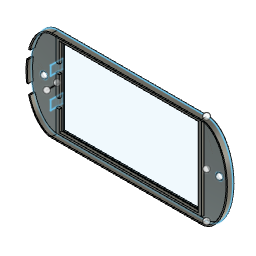
SolarPanelFront_v1 (Autodesk Fusion 360 design; units mm, degrees)
Autodesk Fusion 360 part; units mm, degrees
sketch "Sketch1" plane through (0, 0, 0) normal (0, 1, 0) x (1, 0, 0)
  line L0 (0, 0) -> (115, 0)
  line L1 (115, -70) -> (0, -70)
  ellipse E0 centre (0, -35) end of major axis (0, -70) minor radius 20 (0, 0) -> (0, -70) ccw
  ellipse E1 centre (115, -35) end of major axis (115, -70) minor radius 20 (115, -70) -> (115, 0) ccw
  circle A0 centre (-10, -35) radius 2.5
  circle A1 centre (125, -35) radius 2.5
  dimension "d1" = 20
  dimension "d2" = 5
  dimension "d3" = 10
  constraint horizontal L0
  constraint horizontal L1
  measures "d2" diameter of A0
  measures "d3" distance of E0.centre A0.centre
extrude "Extrude1" add sketch "Sketch1" along normal blind 1
sketch "Sketch3" plane through (0, 0, 0) normal (0, -1, 0) x (1, 0, 0)
  circle A0 centre (-10, 35) radius 2.5
  circle A1 centre (125, 35) radius 2.5
  ellipse E0 centre (0, 35) end of major axis (0, 70) minor radius 20 (0, 70) -> (0, 0) ccw
  line L0 (0, 0) -> (115, 0)
  ellipse E1 centre (115, 35) end of major axis (115, 70) minor radius 20 (115, 0) -> (115, 70) ccw
  line L1 (115, 70) -> (0, 70)
  line L2 (0, 1) -> (115, 1)
  spline S0 degree 3 poles (115, 1) (118.1745, 1) (121.3862, 2.4713) (124.2603, 5.3633) (127.2867, 8.4088) (129.8847, 13.0253) (131.6024, 18.5351) (133.5298, 24.7176) (134.3377, 31.9986) (133.8651, 39.0248) (133.4191, 45.6553) (131.8372, 52.0318) (129.4075, 57.0895) (127.2109, 61.662) (124.3332, 65.1363) (121.2436, 67.0835) (119.2133, 68.3631) (117.1029, 69) (115, 69) knots 3.141593 3.141593 3.141593 3.141593 3.663435 3.663435 3.663435 4.212955 4.212955 4.212955 4.82957 4.82957 4.82957 5.411454 5.411454 5.411454 5.937501 5.937501 5.937501 6.283185 6.283185 6.283185 6.283185
  line L3 (115, 69) -> (0, 69)
  spline S1 degree 3 poles (0, 69) (-3.1745, 69) (-6.3862, 67.5287) (-9.2603, 64.6367) (-12.2867, 61.5912) (-14.8847, 56.9747) (-16.6024, 51.4649) (-18.5298, 45.2824) (-19.3377, 38.0014) (-18.8651, 30.9752) (-18.4191, 24.3447) (-16.8372, 17.9682) (-14.4075, 12.9105) (-12.2109, 8.338) (-9.3332, 4.8637) (-6.2436, 2.9165) (-4.2133, 1.6369) (-2.1029, 1) (0, 1) knots 0 0 0 0 0.521842 0.521842 0.521842 1.071362 1.071362 1.071362 1.687978 1.687978 1.687978 2.269861 2.269861 2.269861 2.795908 2.795908 2.795908 3.141593 3.141593 3.141593 3.141593
  dimension "d6" = -1
extrude "Extrude2" add sketch "Sketch3" along normal blind 4 contours E0 L0 E1 L1
sketch "Sketch4" plane through (0, 0, 0) normal (0, 1, 0) x (1, 0, 0)
  line L0 (3.55, -65.5) -> (110.65, -65.5)
  line L1 (110.65, -65.5) -> (110.65, -4.5)
  line L2 (110.65, -4.5) -> (3.55, -4.5)
  line L3 (3.55, -4.5) -> (3.55, -65.5)
  line L4 (115, -1) -> (0, -1)
  line L5 (1, -67) -> (113, -67)
  line L6 (113, -67) -> (113, -3)
  line L7 (113, -3) -> (1, -3)
  line L8 (1, -3) -> (1, -67)
  point P0 (0, -35)
  dimension "d9" = 61
  dimension "d10" = 107.1
  dimension "d11" = 3.55
  dimension "d12" = 3.5
  constraint horizontal L0
  constraint vertical L1
  constraint horizontal L2
  constraint vertical L3
  constraint horizontal L5
  constraint vertical L6
  constraint horizontal L7
  constraint vertical L8
  measures "d9" distance of L0.start L2.end
  measures "d10" distance of L0.start L0.end
  measures "d11" distance of L3 P0
  measures "d12" distance of L2 L4
extrude "Extrude3" add sketch "Sketch4" against normal blind 2
sketch "Sketch5" plane through (0, 0, 0) normal (0, 1, 0) x (-1, 0, 0)
  line L0 (-4.5848, 64.4333) -> (-109.4505, 64.4333)
  line L1 (-109.4505, 64.4333) -> (-109.4505, 5.2457)
  line L2 (-109.4505, 5.2457) -> (-4.5848, 5.2457)
  line L3 (-4.5848, 5.2457) -> (-4.5848, 64.4333)
  constraint horizontal L0
  constraint vertical L1
  constraint horizontal L2
  constraint vertical L3
extrude "Extrude4" cut sketch "Sketch5" along normal blind 10
sketch "Sketch6" plane through (1, 0, 0) normal (-1, 0, 0) x (0, -1, 0)
  line L0 (0, 67) -> (0, 3)
  line L1 (0, 3) -> (2, 3)
  line L2 (2, 3) -> (2, 67)
  line L3 (2, 67) -> (0, 67)
  line L4 (-3, 27) -> (6, 27)
  line L5 (6, 27) -> (6, 20)
  line L6 (6, 20) -> (-3, 20)
  line L7 (-3, 20) -> (-3, 27)
  line L8 (0, 35) -> (9, 35)
  line L9 (-3, 43) -> (6, 43)
  line L10 (6, 43) -> (6, 50)
  line L11 (6, 50) -> (-3, 50)
  line L12 (-3, 50) -> (-3, 43)
  constraint horizontal L4
  constraint vertical L5
  constraint horizontal L6
  constraint vertical L7
  constraint midpoint L0 L8.start
  constraint perpendicular L2 L8
  constraint symmetric L4.start L8 L9.start
  constraint symmetric L4.end L8 L9.end
  constraint symmetric L5.end L8 L10.end
  constraint symmetric L6.end L8 L11.end
extrude "Extrude5" cut sketch "Sketch6" along normal blind 30 contours L0 L2 L9 L11 | L2 L9 L10 L11
extrude "Extrude6" cut sketch "Sketch6" against normal blind 9 contours L0 L2 L9 L11 | L2 L9 L10 L11
extrude "Extrude7" cut sketch "Sketch6" along normal blind 30 contours L0 L2 L4 L6 | L2 L4 L5 L6
extrude "Extrude8" cut sketch "Sketch6" against normal blind 10 contours L0 L2 L4 L6 | L2 L4 L5 L6
